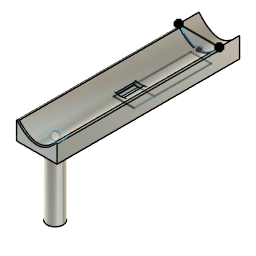
limit_switch_bracket (Autodesk Fusion 360 design; units mm, degrees)
Autodesk Fusion 360 part; units mm, degrees
sketch "Sketch1" plane through (0, 0, 0) normal (0, 0, 1) x (1, 0, 0)
  line L0 (0, 0) -> (-10, 0)
  line L1 (-10, 0) -> (-10, -40)
  line L2 (-10, -40) -> (0, -40)
  line L3 (0, -40) -> (0, 0)
  dimension "d1" = 10
  dimension "d2" = 40
  constraint horizontal L0
  constraint vertical L1
  constraint horizontal L2
  constraint vertical L3
  constraint coincident L0.start L3.end
  measures "d1" distance of L0.start L0.end
  measures "d2" distance of L0.start L2.end
extrude "Extrude1" add sketch "Sketch1" along normal blind 4
sketch "Sketch2" plane through (0, 0, 0) normal (0, 0, -1) x (1, 0, 0)
  line L0 (0, 0) -> (0, 40)
  line L1 (0, 40) -> (-10, 40)
  line L2 (-10, 40) -> (-10, 0)
  line L3 (-10, 0) -> (0, 0)
  circle A0 centre (-5.29, 35.1764) radius 2
  dimension "d5" = 4
  measures "d5" diameter of A0
extrude "Extrude2" add sketch "Sketch2" along normal blind 18 contours A0
sketch "Sketch3" plane through (0, 0, 0) normal (0, 1, 0) x (-1, 0, 0)
  line L0 (0, 0) -> (10, 0)
  line L1 (10, 0) -> (10, 4)
  line L2 (10, 4) -> (0, 4)
  line L3 (0, 4) -> (0, 0)
  spline S0 degree 5 poles (0, 4) (0.2, 3.7624) (0.6, 3.3081) (1.2, 2.6888) (2, 1.9895) (3, 1.3407) (4, 0.9372) (5, 0.7991) (6, 0.9372) (7, 1.3407) (8, 1.9895) (8.8, 2.6888) (9.4, 3.3081) (9.8, 3.7624) (10, 4) knots 0 0 0 0 0 0 0.1 0.2 0.3 0.4 0.5 0.6 0.7 0.8 0.9 1 1 1 1 1 1
  line L4 (0, 4) -> (10, 4)
  point P0 (5, 0.868)
  constraint coincident L2.end L3.start
  constraint coincident L1.end L2.start
extrude "Extrude3" cut sketch "Sketch3" against normal blind 40 contours L2 S0 L4
fillet "Fillet1" radius 0.25 4 edges at (0, -20, 4) (-10, -20, 4) (-5, -40, 0.868) (-5, 0, 0.868)
sketch "Sketch4" plane through (0, 0, 0) normal (0, 0, -1) x (1, 0, 0)
  circle A0 centre (-5.29, 35.1764) radius 2
  line L0 (0, 0) -> (0, 40)
  line L1 (0, 40) -> (-10, 40)
  line L2 (-10, 40) -> (-10, 0)
  line L3 (-10, 0) -> (0, 0)
  line L4 (-6.5, 19.5) -> (-1.5, 19.5)
  line L5 (-1.5, 19.5) -> (-1.5, 0.5)
  line L6 (-1.5, 0.5) -> (-6.5, 0.5)
  line L7 (-6.5, 0.5) -> (-6.5, 19.5)
  line L8 (-6.5, 19.5) -> (-1.5, 19.5)
  line L9 (-1.5, 19.5) -> (-1.5, 14.5)
  line L10 (-1.5, 14.5) -> (-6.5, 14.5)
  line L11 (-6.5, 14.5) -> (-6.5, 19.5)
  dimension "d12" = 5
  dimension "d13" = 19
  dimension "d15" = 19.5
  dimension "d16" = 3.5
  dimension "d23" = 5
  constraint horizontal L4
  constraint vertical L5
  constraint horizontal L6
  constraint vertical L7
  constraint horizontal L8
  constraint vertical L9
  constraint horizontal L10
  constraint vertical L11
  measures "d12" distance of L4.start L4.end
  measures "d13" distance of L4.start L6.end
  measures "d15" distance of L3 L4
  measures "d16" distance of L2 L7
  measures "d23" distance of L4.start L10.end
extrude "Extrude5" add sketch "Sketch4" along normal blind 1
extrude "Extrude6" add sketch "Sketch3" 1 faces at (-5.0081, 0, -0.4607) along normal blind 5 contours L0 L1 L3 S0
extrude "Extrude7" cut sketch "Sketch4" against normal blind 1 contours L4 L5 L7 L8 L9 L10 L11
